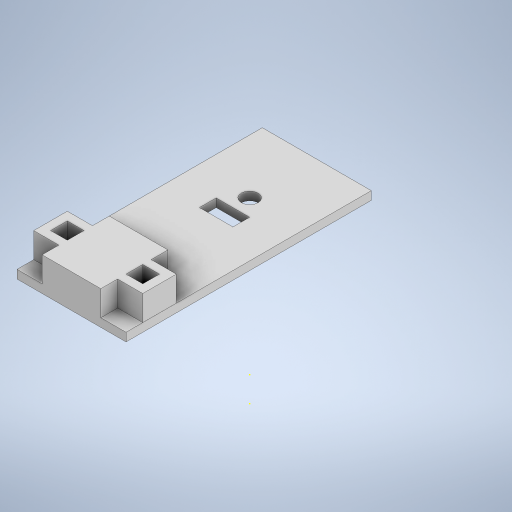
# Autodesk Inventor part: platform
Saved by Autodesk Inventor 2024 (Build 280153000, 153)
## iProperties
Created: 2024-01-23
Part Number: platform
Material: Generic
Document SubType Name: Modeling
Designer: emosh
Density: 1 g/cm^3
Appearance: Default
Author: emosh
## iProperties of the stored document platform_3DPrint.ipt
Created: 2024-01-24
Part Number: platform_3DPrint
Material: Generic
Document SubType Name: Modeling
Designer: emosh
Density: 1 g/cm^3
Appearance: Default
Author: emosh
Autodesk Inventor part; units mm, degrees
ref_plane "YZ Plane" through (0, 0, 0) normal (1, 0, 0) x (0, 1, 0)
ref_plane "XZ Plane" through (0, 0, 0) normal (0, 1, 0) x (-1, 0, 0)
ref_plane "XY Plane" through (0, 0, 0) normal (0, 0, 1) x (1, 0, 0)
sketch "Sketch1" plane through (0, 0, 0) normal (0, 1, 0) x (-1, 0, 0)
  line L0 (46.8313, 0) -> (88.1062, 0)
  line L1 (88.1062, -134.9375) -> (46.8313, -134.9375)
  line L2 (88.1062, -134.9375) -> (67.4688, -134.9375)
  line L3 (67.4688, -134.9375) -> (67.4688, 0)
  line L4 (67.4688, 0) -> (134.9375, 0)
  line L5 (67.4688, -134.9375) -> (78.5812, -134.9375)
  line L6 (78.5812, -134.9375) -> (78.5812, 0)
  line L7 (78.5812, 0) -> (67.4688, 0)
  line L8 (67.4688, 0) -> (67.4688, -134.9375)
  line L9 (78.5812, -134.9375) -> (88.1062, -134.9375)
  line L10 (88.1062, -134.9375) -> (88.1062, 0)
  line L11 (88.1062, 0) -> (78.5812, 0)
  line L12 (78.5812, 0) -> (78.5812, -134.9375)
  line L13 (67.4688, -134.9375) -> (56.3563, -134.9375)
  line L14 (56.3563, -134.9375) -> (56.3563, 0)
  line L15 (56.3563, 0) -> (67.4688, 0)
  line L16 (67.4688, 0) -> (67.4688, -134.9375)
  line L17 (56.3563, 0) -> (46.8313, 0)
  line L18 (46.8313, 0) -> (46.8313, -134.9375)
  line L19 (46.8313, -134.9375) -> (56.3563, -134.9375)
  line L20 (56.3563, -134.9375) -> (56.3563, 0)
  line L21 (88.1062, 0) -> (46.8313, 0)
  line L22 (46.8313, 0) -> (46.8313, -67.4688)
  line L23 (46.8313, -67.4688) -> (88.1062, -67.4688)
  line L24 (88.1062, -67.4688) -> (88.1062, 0)
  line L25 (78.5813, -67.4688) -> (56.3563, -67.4688)
  line L26 (56.3563, -67.4688) -> (56.3563, -92.8688)
  line L27 (56.3563, -92.8688) -> (78.5813, -92.8688)
  line L28 (78.5813, -92.8688) -> (78.5813, -67.4688)
  line L29 (78.5813, -92.8688) -> (88.1062, -92.8688)
  line L30 (56.3563, -92.8688) -> (46.8313, -92.8688)
  dimension "d34" = 11.1125
  dimension "d35" = 9.525
  dimension "d36" = 11.1125
  dimension "d53" = 9.525
  dimension "d54" = 25.4
  constraints: 62 end point, 14 parallel, 8 horizontal, 8 perpendicular, 8 point on line, 3 midpoint
  measures "d34" distance of L7.end L6.end
  measures "d35" distance of L0.end L11.end
  measures "d36" distance of L14.end L15.end
  measures "d53" distance of L0.start L14.end
  measures "d54" distance of L26.end L25.end
extrude "Extrusion1" add sketch "Sketch1" along normal blind 3.175 contours L0 L14 L23 L18 | L0 L3 L23 L14 | L23 L14 L30 L18 | L0 L6 L23 L3 | L23 L3 L27 L14 | L0 L10 L23 L6 | L23 L6 L27 L3 | L23 L10 L29 L6
sketch "Sketch2" plane through (0, 3.175, 0) normal (0, 1, 0) x (1, 0, 0)
  line L0 (0, 0) -> (0, 134.9375) projected
  line L1 (0, 0) -> (-57.15, 0)
  line L2 (-57.15, 0) -> (-68.2625, 0)
  line L3 (-57.15, 0) -> (-67.4751, 0)
  line L4 (-57.15, 0) -> (-79.375, 0)
  line L5 (-67.4751, 25.4) -> (-57.15, 25.4)
  line L6 (-67.4751, 25.4) -> (-56.3626, 25.4)
  line L7 (-56.3626, 25.4) -> (-56.3626, 0)
  line L8 (-56.3626, 0) -> (-67.4751, 0)
  line L9 (-67.4751, 0) -> (-67.4751, 25.4)
  line L10 (-67.4751, 0) -> (-78.5876, 0)
  line L11 (-78.5876, 0) -> (-78.5876, 25.4)
  line L12 (-78.5876, 25.4) -> (-67.4751, 25.4)
  line L13 (-67.4751, 25.4) -> (-67.4751, 0)
  point P0 (-46.8313, 134.9375)
  point P1 (-67.4751, 0)
  point P2 (-68.2625, 0)
  dimension "d39" = 11.1125
  dimension "d40" = 25.4
  dimension "d41" = 11.1125
  dimension "d42" = 25.4
  constraints: 26 end point, 5 horizontal, 5 parallel, 2 perpendicular, 1 point on line
  measures "d39" distance of L7.end L8.end
  measures "d40" distance of L6.end L7.end
  measures "d41" distance of L11.end L12.end
  measures "d42" distance of L10.end L11.end
extrude "Extrusion2" add sketch "Sketch2" along normal blind 9.525
sketch "Sketch3" plane through (0, 3.175, 0) normal (0, 1, 0) x (1, 0, 0)
  line L0 (0, 0) -> (-67.4751, 0)
  line L1 (-67.4751, 0) -> (-67.4751, 67.4751)
  line L2 (-67.4751, 67.4751) -> (0, 67.4751)
  line L3 (0, 67.4751) -> (0, 0)
  circle A0 centre (-67.4751, 67.4751) radius 3.175
  dimension "d13" = 67.4751
  dimension "d14" = 67.4751
  dimension "d15" = 6.35
  constraints: 8 end point, 2 parallel, 1 centre point, 1 coincident, 1 horizontal, 1 perpendicular
  measures "d13" distance of L1.end L2.end
  measures "d14" distance of L0.end L1.end
  measures "d15" diameter of A0
extrude "Extrusion3" cut sketch "Sketch3" against normal blind 6.35 contours A0 L2 L1 | L1 L2 A0
sketch "Sketch4" plane through (0, 12.7, 0) normal (0, 1, 0) x (1, 0, 0)
  point P0 (0, 0)
sketch "Sketch5" plane through (0, 3.175, 0) normal (0, 1, 0) x (1, 0, 0)
  line L0 (-56.3626, 0) -> (0, 0) projected
  line L1 (0, 0) -> (-67.4751, 0)
  line L2 (-67.4751, 0) -> (-67.4751, 67.4751)
  line L3 (-67.4751, 67.4751) -> (0, 67.4751)
  line L4 (0, 67.4751) -> (0, 0)
  line L5 (-56.3626, 25.4) -> (-78.5876, 25.4) projected
  line L6 (-56.3626, 0) -> (-56.3626, 25.4) projected
  line L7 (-67.4751, 25.4) -> (-56.3626, 25.4)
  line L8 (-56.3626, 25.4) -> (-56.3626, 12.7)
  line L9 (-56.3626, 12.7) -> (-67.4751, 12.7)
  line L10 (-67.4751, 12.7) -> (-67.4751, 25.4)
  line L11 (-50.0126, 12.7) -> (-50.0126, 19.05)
  line L12 (-50.0126, 19.05) -> (-56.3626, 19.05)
  line L13 (-56.3626, 19.05) -> (-56.3626, 12.7)
  line L14 (-50.0126, 12.7) -> (-50.0126, 6.35)
  line L15 (-50.0126, 6.35) -> (-56.3626, 6.35)
  line L16 (-56.3626, 6.35) -> (-56.3626, 12.7)
  line L17 (-56.3626, 19.05) -> (-50.0126, 19.05)
  line L18 (-50.0126, 19.05) -> (-50.0126, 15.875)
  line L19 (-50.0126, 15.875) -> (-56.3626, 15.875)
  line L20 (-56.3626, 15.875) -> (-56.3626, 19.05)
  line L21 (-56.3626, 6.35) -> (-50.0126, 6.35)
  line L22 (-50.0126, 6.35) -> (-50.0126, 9.525)
  line L23 (-50.0126, 9.525) -> (-56.3626, 9.525)
  line L24 (-56.3626, 9.525) -> (-56.3626, 6.35)
  line L25 (-56.3626, 19.05) -> (-46.8376, 19.05)
  line L26 (-46.8376, 19.05) -> (-46.8376, 6.35)
  line L27 (-46.8376, 6.35) -> (-56.3626, 6.35)
  line L28 (-56.3626, 6.35) -> (-56.3626, 19.05)
  line L29 (-78.5876, 25.4) -> (-78.5876, 0) projected
  line L30 (-78.5876, 19.05) -> (-88.1126, 19.05)
  line L31 (-88.1126, 19.05) -> (-88.1126, 6.35)
  line L32 (-88.1126, 6.35) -> (-78.5876, 6.35)
  line L33 (-78.5876, 6.35) -> (-78.5876, 19.05)
  line L34 (-88.1126, 19.05) -> (-84.9376, 19.05)
  line L35 (-84.9376, 19.05) -> (-84.9376, 6.35)
  line L36 (-84.9376, 6.35) -> (-88.1126, 6.35)
  line L37 (-88.1126, 6.35) -> (-88.1126, 19.05)
  line L38 (-84.9376, 15.875) -> (-78.5876, 15.875)
  line L39 (-78.5876, 15.875) -> (-78.5876, 9.525)
  line L40 (-78.5876, 9.525) -> (-84.9376, 9.525)
  line L41 (-84.9376, 9.525) -> (-84.9376, 15.875)
  point P0 (-57.15, 25.4)
  point P1 (-57.15, 0)
  point P2 (-79.375, 0)
  dimension "d43" = 67.4751
  dimension "d44" = 67.4751
  dimension "d46" = 6.35
  dimension "d49" = 9.525
  dimension "d50" = 9.525
  dimension "d51" = 3.175
  constraints: 76 end point, 18 parallel, 8 horizontal, 8 perpendicular, 4 midpoint, 4 point on line
  measures "d43" distance of L2.end L3.end
  measures "d44" distance of L1.end L2.end
  measures "d46" distance of L12.end L11.end
  measures "d49" distance of L26.end L27.end
  measures "d50" distance of L32.end L31.end
  measures "d51" distance of L35.end L36.end
extrude "Extrusion4" add sketch "Sketch5" along normal blind 9.525 contours L29 L38 L35 L30 | L6 L23 L14 L15 | L14 L11 L25 L26 L27 | L6 L12 L11 L19 | L35 L32 L31 L30 | L29 L32 L35 L40
sketch "Sketch6" plane through (0, 3.175, 0) normal (0, 1, 0) x (1, 0, 0)
  point P0 (0, 0)
sketch "Sketch7" plane through (0, 3.175, 0) normal (0, 1, 0) x (1, 0, 0)
  line L0 (-46.8313, 92.8688) -> (-88.1062, 92.8688) projected
  line L1 (-46.8313, 0) -> (-46.8313, 92.8688) projected
  line L2 (-88.1062, 92.8688) -> (-46.8313, 92.8688)
  line L3 (-46.8313, 92.8688) -> (-46.8313, 67.4688)
  line L4 (-46.8313, 67.4688) -> (-88.1062, 67.4688)
  line L5 (-88.1062, 67.4688) -> (-88.1062, 92.8688)
  line L6 (-88.1062, 67.4688) -> (-67.4687, 67.4688)
  line L7 (-67.4687, 67.4688) -> (-67.4687, 42.0688)
  line L8 (-67.4687, 42.0688) -> (-88.1062, 42.0688)
  line L9 (-88.1062, 42.0688) -> (-88.1062, 67.4688)
  line L10 (-67.4687, 42.0688) -> (-73.8187, 42.0688)
  line L11 (-73.8187, 42.0688) -> (-73.8187, 61.1188)
  line L12 (-73.8187, 61.1188) -> (-67.4687, 61.1188)
  line L13 (-67.4687, 61.1188) -> (-67.4687, 42.0688)
  line L14 (-73.8187, 61.1188) -> (-61.1187, 61.1188)
  line L15 (-61.1187, 61.1188) -> (-61.1187, 54.7687)
  line L16 (-61.1187, 54.7687) -> (-73.8187, 54.7687)
  line L17 (-73.8187, 54.7687) -> (-73.8187, 61.1188)
  point P0 (0, 0)
  dimension "d55" = 25.4
  dimension "d56" = 20.6375
  dimension "d57" = 25.4
  dimension "d58" = 6.35
  dimension "d59" = 19.05
  dimension "d60" = 12.7
  constraints: 32 end point, 8 parallel, 4 horizontal, 4 perpendicular, 1 coincident, 1 point on line
  measures "d55" distance of L2.end L3.end
  measures "d56" distance of L7.end L8.end
  measures "d57" distance of L6.end L7.end
  measures "d58" distance of L11.end L12.end
  measures "d59" distance of L10.end L11.end
  measures "d60" distance of L15.end L16.end
extrude "Extrusion5" cut sketch "Sketch7" against normal blind 25.4 contours L14 L15 L16 L7 | L7 L16 L11 L12
body "Solid1"
